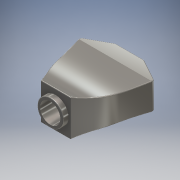
# Autodesk Inventor part: Cabeça da tarraxa
Saved by Autodesk Inventor 2016 (Build 200138000, 138)
## iProperties
Created: 2018-12-04
Part Number: Cabeça da tarraxa
Material: Generic
Document SubType Name: Sheet Metal
Designer: dqm_r
Density: 1 g/cm^3
Sheet Metal Rule: Default_mm
Appearance: Steel - Polished
Author: dqm_r
Autodesk Inventor part; units mm, degrees
ref_plane "YZ Plane" through (0, 0, 0) normal (1, 0, 0) x (0, 1, 0)
ref_plane "XZ Plane" through (0, 0, 0) normal (0, 1, 0) x (-1, 0, 0)
ref_plane "XY Plane" through (0, 0, 0) normal (0, 0, 1) x (1, 0, 0)
sketch "Sketch3" plane through (0, 0, 0) normal (0, 0, 1) x (1, 0, 0)
  line L0 (-9.4, -9.4) -> (9.4, -9.4)
  line L1 (9.4, -9.4) -> (9.4, 9.4)
  line L2 (9.4, 9.4) -> (-9.4, 9.4)
  line L3 (-9.4, 9.4) -> (-9.4, -9.4)
  line L4 (-9.4, -9.4) -> (9.4, 9.4) construction
  line L5 (9.4, -9.4) -> (-9.4, 9.4) construction
  point P0 (0, 0)
  dimension "d2" = 18.8
  dimension "d3" = 18.8
  constraints: 12 end point, 2 midpoint, 2 parallel, 1 horizontal, 1 perpendicular
  measures "d2" distance of L0.start L0.end
  measures "d3" distance of L1.end L0.end
extrude "Extrusion1" add sketch "Sketch3" along normal blind 9.4
sketch "Sketch5" plane through (0, 0, 9.4) normal (0, 0, 1) x (1, 0, 0)
  line L0 (9.4, 9.4) -> (-9.4, 9.4) projected
  line L1 (-9.4, 9.4) -> (-9.4, 6.2)
  line L2 (-9.4, 9.4) -> (-9.4, -9.4) projected
  line L3 (-9.4, 9.4) -> (-3.6, 9.4)
  line L4 (-9.4, 6.2) -> (-3.6, 9.4)
  line L5 (9.4, 9.4) -> (3.6, 9.4)
  line L6 (3.6, 9.4) -> (9.4, 6.2)
  line L7 (9.4, -9.4) -> (9.4, 9.4) projected
  line L8 (9.4, 9.4) -> (9.4, 6.2)
  line L9 (-9.4, 6.2) -> (-9.4, -9.4)
  line L10 (9.4, 6.2) -> (9.4, -9.4)
  line L11 (9.4, -9.4) -> (9.4, -3.4)
  line L12 (9.4, 6.2) -> (7, -3.4)
  line L13 (3.74, -9.4) -> (7, -3.4)
  line L14 (-9.4, 6.2) -> (-7, -3.4)
  line L15 (-7, -3.4) -> (-3.74, -9.4)
  line L16 (3.74, -9.4) -> (9.4, -9.4)
  line L17 (-3.74, -9.4) -> (-9.4, -9.4)
  point P0 (0, 0)
  point P1 (0, -9.4)
  point P2 (0, -3.4)
  point P3 (0, -9.4)
  point P4 (0, -9.4)
  point P5 (0, -3.4)
  dimension "d7" = 3.2
  dimension "d8" = 5.8
  dimension "d9" = 5.8
  dimension "d22" = 7.48
  dimension "d23" = 14
  constraints: 30 end point, 5 point on line, 2 collinear, 1 coincident, 1 horizontal
  measures "d7" distance of L0.end L1.end
  measures "d8" distance of L0.end L3.end
  measures "d9" distance of L0.start L5.end
  measures "d22" distance of L15.end L13.start
  measures "d23" distance of L12.end L14.end
extrude "Extrusion2" cut sketch "Sketch5" against normal blind 9.4
fillet "Fillet3" radius 0.7 2 edges at (3.6, 9.4, 4.7) (-3.6, 9.4, 4.7)
fillet "Fillet4" radius 20 1 edges at (7, -3.4, 4.7)
fillet "Fillet6" radius 20 1 edges at (-7, -3.4, 4.7)
fillet "Fillet7" radius 0.7 1 edges at (-9.4, 6.2, 4.7)
fillet "Fillet8" radius 0.7 1 edges at (9.4, 6.2, 4.7)
sketch "Sketch6" plane through (0, 0, 0) normal (1, 0, 0) x (0, 1, 0)
  line L0 (-9.4, 9.4) -> (-5.6326, 9.4) projected
  line L1 (5.6775, 9.4) -> (6.4602, 9.4) projected
  line L2 (5.6775, 8.1) -> (0.9541, 7.7565) construction
  line L3 (0.9541, 7.7565) -> (-5.2928, 7.7565) construction
  line L4 (-5.2928, 7.7565) -> (-9.4, 9.4) construction
  spline S0 degree 3 poles (5.6775, 8.1) (0.9541, 7.7565) (-5.2928, 7.7565) (-9.4, 9.4) knots 1 1 1 1 2 2 2 2
  line L5 (-9.4, 9.4) -> (-9.4, 0) projected
  line L6 (-9.4, 4.7) -> (-6.9868, 4.7) construction
  line L7 (5.6775, 1.3) -> (0.9541, 1.6435) construction
  line L8 (0.9541, 1.6435) -> (-5.2928, 1.6435) construction
  line L9 (-5.2928, 1.6435) -> (-9.4, 0) construction
  spline S1 degree 3 poles (5.6775, 1.3) (0.9541, 1.6435) (-5.2928, 1.6435) (-9.4, 0) knots 1 1 1 1 2 2 2 2
  line L10 (5.6775, 8.1) -> (9.4, 8.1)
  line L11 (6.4602, 9.4) -> (9.3129, 9.4) projected
  line L12 (-9.4, 0) -> (9.3129, 0)
  line L13 (5.6775, 1.3) -> (9.3129, 1.3)
  line L14 (9.4, 8.1) -> (9.4, 9.4)
  line L15 (9.3129, 9.4) -> (9.3129, 0) projected
  line L16 (9.4, 9.4) -> (-9.4, 9.4)
  line L17 (9.3129, 1.3) -> (9.8669, 1.3)
  line L18 (9.8669, 1.3) -> (9.8669, 0)
  line L19 (9.4, 0) -> (9.3129, 0) projected
  line L20 (9.8669, 0) -> (9.3129, 0)
  point P0 (0, 0)
  point P1 (6.0688, 9.4)
  constraints: 18 end point, 3 symmetric about line, 2 horizontal, 2 midpoint, 2 perpendicular, 1 collinear, 1 parallel, 6 other
extrude "Extrusion3" cut sketch "Sketch6" along normal through all both and the other way through all contours L0 L16 L1 L11 L15 L10 S0 | S1 L13 L15 L12 | L15 L16 L14 L10 | L15 L17 L18 L20 L19
sketch "Sketch7" plane through (-3.4197, 9.4, 1.3) normal (0, 1, 0) x (1, 0, 0)
  line L0 (0, -6.8) -> (6.8394, -6.8) projected
  line L1 (3.4197, -6.8) -> (3.4197, 0)
  line L2 (6.8394, 0) -> (0, 0) projected
  circle A0 centre (3.4197, -3.4) radius 1.0441
  point P0 (3.4197, 1.3)
  constraints: 3 midpoint, 2 end point, 1 centre point
sketch "Sketch8" plane through (-3.74, -9.4, 9.4) normal (0, -1, 0) x (1, 0, 0)
  line L0 (3.74, -9.4) -> (3.74, 0) construction
  line L1 (0, 0) -> (7.48, 0) projected
  circle A0 centre (3.74, -4.7) radius 3.3
  circle A1 centre (3.74, -4.7) radius 2.57
  dimension "d30" = 6.6
  dimension "d31" = 5.14
  constraints: 2 centre point, 2 end point, 2 midpoint, 1 coincident
  measures "d30" diameter of A0
  measures "d31" diameter of A1
extrude "Extrusion4" add sketch "Sketch8" along normal blind 1.34
hole "Hole1" at (0, 9.4, 4.7) direction (0, -1, 0) diameter 3 depth 7.8 tip angle 118
sketch "Sketch9" plane through (0, -9.4, 4.7) normal (0, -1, 0) x (1, 0, 0)
  circle A0 centre (0, 0) radius 1.7692
  point P0 (0, -4.7)
  constraints: 1 centre point
hole "Hole2" at (0, -9.4, 4.7) direction (0, 1, 0) diameter 5.14 depth 11 tip angle 118
chamfer "Chamfer1" distance 1 angle 45 1 edges at (0, 9.4, 3.2)
fillet "Fillet9" radius 0.2 6 edges at (1.87, -9.4, 0) (-1.87, -9.4, 0) (3.74, -9.4, 4.7) (-1.87, -9.4, 9.4) (1.87, -9.4, 9.4) (-3.74, -9.4, 4.7)
fillet "Fillet10" radius 0.2 32 edges at (6.8315, -3.3896, 8.105) (4.8293, -7.3952, 8.7608) (3.8439, -9.2089, 9.3079) (3.7186, -9.3746, 9.2057) (8.4433, 2.3733, 7.9369) (6.8315, -3.3896, 1.295) (4.8293, -7.3952, 0.6392) (3.8439, -9.2089, 0.0921) (3.7186, -9.3746, 0.1943) (8.4433, 2.3733, 1.4631) (-6.8315, -3.3896, 1.295) (-4.8293, -7.3952, 0.6392) (-3.8439, -9.2089, 0.0921) (-3.7186, -9.3746, 0.1943) (-8.4433, 2.3733, 1.4631) (-6.8315, -3.3896, 8.105) (-4.8293, -7.3952, 8.7608) (-3.8439, -9.2089, 9.3079) (-3.7186, -9.3746, 9.2057) (-8.4433, 2.3733, 7.9369) (3.5943, 9.3779, 8.1) (6.3431, 7.8865, 8.1) (9.232, 6.1268, 8.1) (-3.5943, 9.3779, 8.1) (-6.3431, 7.8865, 8.1) (-9.232, 6.1268, 8.1) (0, 9.4, 8.1) (-6.3431, 7.8865, 1.3) (-9.232, 6.1268, 1.3) (6.3431, 7.8865, 1.3) (9.232, 6.1268, 1.3) (-3.3, -10.74, 4.7)
equation "\"BendRadius\" = Thickness"
equation "\"BendReliefWidth\" = Thickness"
equation "\"BendReliefDepth\" = 0.5 * Thickness"
equation "\"CornerReliefSize\" = 4 * Thickness"
equation "\"MinimumRemnant\" = 2 * Thickness"
equation "\"TransitionRadius\" = BendRadius"
equation "\"JacobiRadiusSize\" = BendRadius"
equation "\"GapSize\" = Thickness"
equation "\"Thickness\" = 0.5"
body "Solid1"
